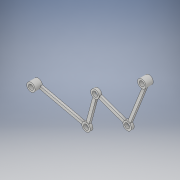
# Autodesk Inventor part: MassiveGearHOlder
Saved by Autodesk Inventor 2017 (Build 210142000, 142)
## iProperties
Created: 2020-09-10
Part Number: MassiveGearHOlder
Material: Generic
Document SubType Name: Modeling
Designer: agustin
Density: 1 g/cm^3
Appearance: Default
Author: agustin
## iProperties of the stored document gear-holder_3DPrint.ipt
Created: 2021-01-25
Part Number: gear-holder_3DPrint
Material: Generic
Document SubType Name: Modeling
Designer: agustin
Density: 1 g/cm^3
Appearance: Default
Author: agustin
Autodesk Inventor part; units mm, degrees
ref_plane "YZ Plane" through (0, 0, 0) normal (1, 0, 0) x (0, 1, 0)
ref_plane "XZ Plane" through (0, 0, 0) normal (0, 1, 0) x (-1, 0, 0)
ref_plane "XY Plane" through (0, 0, 0) normal (0, 0, 1) x (1, 0, 0)
sketch "Sketch1" plane through (0, 0, 0) normal (0, 0, 1) x (1, 0, 0)
  line L0 (125.272, 1.0352) -> (94.9914, -14.9276) projected
  arc A0 (97.3229, -19.3507) -> (94.9914, -14.9276) centre (89.9019, -20.4364) ccw projected
  line L1 (97.3229, -19.3507) -> (127.6037, -3.3892) projected
  line L2 (157.89, 12.5592) -> (127.6037, -3.3892) projected
  arc A1 (155.5603, 16.9833) -> (157.89, 12.5592) centre (162.9818, 18.0659) ccw projected
  line L3 (125.272, 1.0352) -> (155.5603, 16.9833) projected
  circle A2 centre (162.9818, 18.0659) radius 4.5 projected
  circle A3 centre (162.9818, 18.0659) radius 7.5 projected
  arc A4 (192.0328, 98.1186) -> (196.6808, 96.2757) centre (196.9631, 103.7704) ccw projected
  line L4 (163.264, 25.5606) -> (192.0328, 98.1186) projected
  arc A5 (167.912, 23.7177) -> (163.264, 25.5606) centre (162.9818, 18.0659) ccw projected
  line L5 (196.6808, 96.2757) -> (167.912, 23.7177) projected
  circle A6 centre (196.9631, 103.7704) radius 4.5 projected
  circle A7 centre (196.9631, 103.7704) radius 7.5 projected
  circle A8 centre (89.9019, -20.4364) radius 4.5 projected
  circle A9 centre (89.9019, -20.4364) radius 7.5 projected
  arc A10 (6.341, -4.0052) -> (7.4493, 0.8704) centre (0, 0) ccw projected
  line L6 (6.341, -4.0052) -> (82.4526, -21.3068) projected
  arc A11 (83.5609, -16.4312) -> (82.4526, -21.3068) centre (89.9019, -20.4364) ccw projected
  line L7 (83.5609, -16.4312) -> (7.4493, 0.8704) projected
  circle A12 centre (0, 0) radius 4.5 projected
  circle A13 centre (0, 0) radius 7.5 projected
  circle A14 centre (105.6859, 38.2113) radius 3.464 construction
  circle A15 centre (101.9441, 45.313) radius 4.5 construction
  arc A16 (109.4545, 45.313) -> (97.6972, 39.1186) centre (101.9441, 45.313) ccw construction
  circle A17 centre (105.6859, 38.2113) radius 4.5
  line L8 (111.3563, 33.3025) -> (155.487, 17.786)
  arc A18 (106.528, 30.7587) -> (111.3563, 33.3025) centre (105.6859, 38.2113) ccw
  arc A19 (113.1807, 38.4912) -> (101.217, 32.1881) centre (105.6859, 38.2113) ccw
  line L9 (157.3113, 22.9747) -> (113.1807, 38.4912)
  line L10 (163.0842, 20.9449) -> (163.0574, 20.9543)
  line L11 (101.217, 32.1881) -> (89.0598, -12.9838)
  line L12 (94.3708, -14.4132) -> (106.528, 30.7587)
  point P0 (0, 0)
  point P1 (97.7939, 8.8875)
  point P2 (134.3338, 28.1386)
  dimension "d0" = 9
  dimension "d2" = 7.5104
  dimension "d5" = 0.002
  constraints: 10 end point, 8 point on circle, 3 centre point, 3 parallel, 2 coincident, 2 point on line
  measures "d0" diameter of A15
  measures "d2" radius of A16
  measures "d5" angle of L1 L0
extrude "Extrusion1" add sketch "Sketch1" along normal blind 4 contours A0 A9 | A3 A1 | A9 L11 A19 L9 A3 L8 A18 L12 | L6 A10 L7 A9 | A3 L4 A4 L5 | A13 A10 | A4 A7
sketch "Sketch2" plane through (0, 0, 4) normal (0, 0, 1) x (1, 0, 0)
  circle A0 centre (0, 0) radius 4.5
  circle A1 centre (0, 0) radius 7.5
  circle A2 centre (196.9631, 103.7704) radius 4.5 projected
  circle A3 centre (196.9631, 103.7704) radius 4.5
  circle A4 centre (196.9631, 103.7704) radius 7.5
  constraints: 4 centre point, 4 coincident
extrude "Extrusion2" add sketch "Sketch2" along normal blind 9
sketch "Sketch3" plane through (0, 0, 4) normal (0, 0, 1) x (1, 0, 0)
  circle A0 centre (89.9019, -20.4364) radius 4.5 projected
  circle A1 centre (89.9019, -20.4364) radius 4.5
  circle A2 centre (89.9019, -20.4364) radius 7.5
  circle A3 centre (105.6859, 38.2113) radius 4.5 projected
  circle A4 centre (105.6859, 38.2113) radius 4.5
  circle A5 centre (105.6859, 38.2113) radius 7.5
  circle A6 centre (162.9818, 18.0659) radius 4.5 projected
  circle A7 centre (162.9818, 18.0659) radius 4.5
  circle A8 centre (162.9818, 18.0659) radius 7.5
  point P0 (0, 0)
  constraints: 6 centre point, 6 coincident
extrude "Extrusion3" add sketch "Sketch3" along normal blind 1
scale "Scale1" factors (0.5, 0.5, 0.5) then translate (55.6782, 16.6513, 0) bodies 1
body "Solid1"
